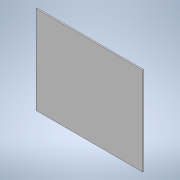
# Autodesk Inventor part: панель_с_электроникой
Saved by Autodesk Inventor 2021.1 (Build 251245010, 245A)
## iProperties
Created: 2023-01-21
Part Number: панель_с_электроникой
Material: Типовые
Document SubType Name: ЛистМат
Designer: zmoze
Density: 1 g/cm^3
Sheet Metal Rule: По умолчанию_мм
Appearance: По умолчанию
Author: zmoze
Autodesk Inventor part; units mm, degrees
ref_plane "YZ Plane" through (0, 0, 0) normal (1, 0, 0) x (0, 1, 0)
ref_plane "XZ Plane" through (0, 0, 0) normal (0, 1, 0) x (-1, 0, 0)
ref_plane "XY Plane" through (0, 0, 0) normal (0, 0, 1) x (1, 0, 0)
sketch "Эскиз1" plane through (0, 0, 0) normal (0, 0, 1) x (1, 0, 0)
  line L0 (-145, 120) -> (145, 120)
  line L1 (145, 120) -> (145, -120)
  line L2 (145, -120) -> (-145, -120)
  line L3 (-145, -120) -> (-145, 120)
  line L4 (-145, 120) -> (145, -120) construction
  line L5 (145, 120) -> (-145, -120) construction
  point P0 (0, 0)
  dimension "d0" = 240
  dimension "d1" = 290
  measures "d0" distance of L2.end L0.start
  measures "d1" distance of L0.start L0.end
extrude "Пластина1" add sketch "Эскиз1" along normal blind 3
equation "\"d2\" = Толщина"
equation "\"Радиус_гибки\" = Толщина"
equation "\"Ширина_просечки\" = Толщина"
equation "\"Глубина_просечки\" = 0.5 * Толщина"
equation "\"Размер_просечки\" = 4 * Толщина"
equation "\"Мин_остаток\" = 2 * Толщина"
equation "\"Радиус_перехода\" = Радиус_гибки"
equation "\"Радиус_Якоби\" = Радиус_гибки"
equation "\"Размер_зазора\" = Толщина"
equation "\"Толщина\" = 3"
